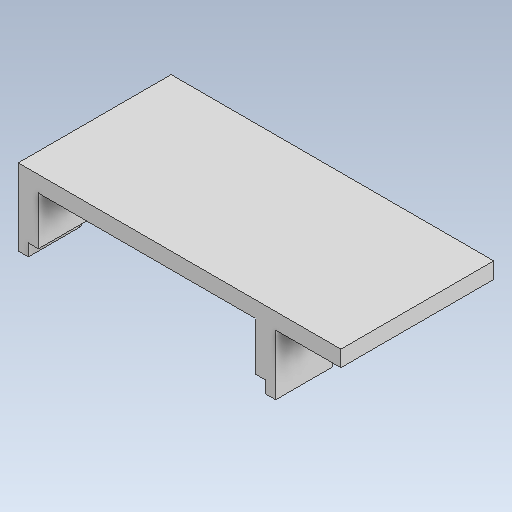
# Autodesk Inventor part: BackPlate
Saved by Autodesk Inventor 2020.1 (Build 241239000, 239)
## iProperties
Created: 2023-01-09
Part Number: BackPlate
Material: Типовые
Document SubType Name: Modeling
Designer: KirikDK
Density: 1 g/cm^3
Appearance: По умолчанию
Author: KirikDK
Autodesk Inventor part; units mm, degrees
ref_plane "YZ Plane" through (0, 0, 0) normal (1, 0, 0) x (0, 1, 0)
ref_plane "XZ Plane" through (0, 0, 0) normal (0, 1, 0) x (-1, 0, 0)
ref_plane "XY Plane" through (0, 0, 0) normal (0, 0, 1) x (1, 0, 0)
sketch "Эскиз1" plane through (0, 0, 0) normal (0, 1, 0) x (-1, 0, 0)
  arc A0 (313.5, 70) -> (307.5, 64) centre (313.5, 64) ccw
  line L0 (307.5, 0) -> (307.5, 64)
  line L1 (320, 0) -> (307.5, 0)
  line L2 (320, 70) -> (320, 0)
  line L3 (313.5, 70) -> (320, 70)
  arc A1 (307.5, 126) -> (313.5, 120) centre (313.5, 126) ccw
  line L4 (320, 120) -> (313.5, 120)
  line L5 (320, 190) -> (320, 120)
  line L6 (307.5, 190) -> (320, 190)
  line L7 (307.5, 126) -> (307.5, 190)
  arc A2 (6.5, 120) -> (12.5, 126) centre (6.5, 126) ccw
  line L8 (12.5, 190) -> (12.5, 126)
  line L9 (0, 190) -> (12.5, 190)
  line L10 (0, 120) -> (0, 190)
  line L11 (6.5, 120) -> (0, 120)
  line L12 (12.5, 64) -> (12.5, 0)
  arc A3 (12.5, 64) -> (6.5, 70) centre (6.5, 64) ccw
  line L13 (0, 70) -> (6.5, 70)
  line L14 (0, 0) -> (0, 70)
  line L15 (12.5, 0) -> (0, 0)
  line L16 (12.5, 64) -> (12.5, 0)
  point P0 (144, 0)
  constraints: 34 end point, 8 point on circle, 4 centre point
extrude "Выдавливание1" add sketch "Эскиз1" along normal blind 15
sketch "Эскиз2" plane through (0, 15, 0) normal (0, 1, 0) x (1, 0, 0)
  line L0 (-320, -120) -> (-320, -190) projected
  line L1 (-320, -190) -> (-295, -190)
  line L2 (-295, -190) -> (-295, 0)
  line L3 (-295, 0) -> (-320, 0)
  line L4 (-320, 0) -> (-320, -190)
  line L5 (0, -190) -> (0, -120) projected
  line L6 (0, -190) -> (-25, -190)
  line L7 (-25, -190) -> (-25, 0)
  line L8 (-25, 0) -> (0, 0)
  line L9 (0, 0) -> (0, -190)
  point P0 (0, 0)
  dimension "d2" = 25
  dimension "d3" = 25
  constraints: 16 end point, 4 parallel, 2 horizontal, 2 perpendicular, 1 point on line
  measures "d2" distance between parallel lines of L4 L2
  measures "d3" distance between parallel lines of L5 L7
extrude "Выдавливание2" add sketch "Эскиз2" along normal blind 60
sketch "Эскиз3" plane through (0, 75, 0) normal (0, 1, 0) x (1, 0, 0)
  line L0 (-320, 0) -> (-320, -190) projected
  line L1 (-320, -190) -> (81, -190)
  line L2 (81, -190) -> (81, 0)
  line L3 (81, 0) -> (-320, 0)
  line L4 (-320, 0) -> (-320, -190)
  point P0 (0, 0)
  constraints: 8 end point, 2 parallel, 1 horizontal, 1 perpendicular
extrude "Выдавливание3" add sketch "Эскиз3" along normal blind 20
